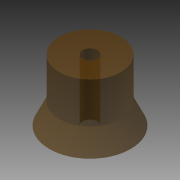
# Autodesk Inventor part: Offset
Saved by Autodesk Inventor 2014 (Build 180170000, 170)
## iProperties
Created: 2014-02-07
Part Number: Offset
Material: Polycarbonate, Smoke
Document SubType Name: Modeling
Designer: Spooner
Density: 1.2 g/cm^3
Appearance: Polycarbonate - Smoked
Mass: 2.0518 g
Surface Area: 10.0971 cm^2
Volume: 1.70984 cm^3
Author: Spooner
Autodesk Inventor part; units mm, degrees
ref_plane "YZ Plane" through (0, 0, 0) normal (1, 0, 0) x (0, 1, 0)
ref_plane "XZ Plane" through (0, 0, 0) normal (0, 1, 0) x (-1, 0, 0)
ref_plane "XY Plane" through (0, 0, 0) normal (0, 0, 1) x (1, 0, 0)
sketch "Sketch1" plane through (0, 0, 0) normal (0, 0, 1) x (1, 0, 0)
  line L0 (8.382, 0) -> (0, 0)
  line L1 (0, 0) -> (0, 12.7)
  line L2 (0, 12.7) -> (6.35, 12.7)
  line L3 (6.35, 12.7) -> (6.35, 4.318)
  line L4 (6.35, 4.318) -> (8.382, 0)
  dimension "d0" = 8.382
  dimension "d1" = 12.7
  dimension "d2" = 8.382
  dimension "d3" = 6.35
  constraints: 10 end point, 2 parallel, 1 horizontal, 1 perpendicular
  measures "d0" distance of L0.start L0.end
  measures "d1" distance of L0.end L1.end
  measures "d2" distance of L2.end L3.end
  measures "d3" distance of L1.end L2.end
revolve "Revolution1" add sketch "Sketch1" angle 360 about axis through (0, 0, 0) along (0, 1, 0)
sketch "Sketch2" plane through (0, 12.7, 0) normal (0, 1, 0) x (1, 0, 0)
  circle A0 centre (0, 0) radius 6.35 projected
  circle A1 centre (0, 0) radius 1.524
  dimension "d5" = 3.048
  constraints: 1 centre point, 1 coincident
  measures "d5" diameter of A1
extrude "Extrusion1" cut sketch "Sketch2" against normal through all contours A1
body "Solid1"
